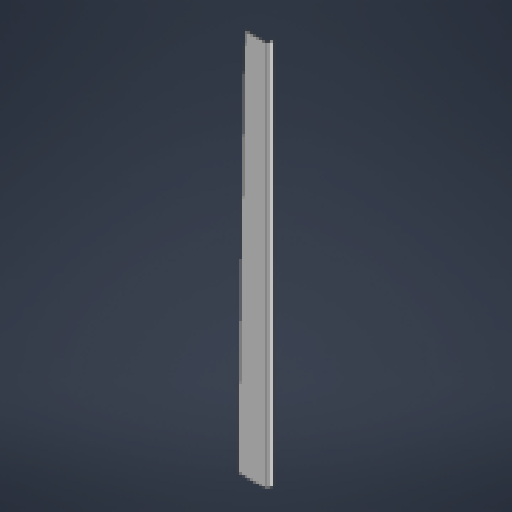
# Autodesk Inventor part: Part2_CPY_CPY
Saved by Autodesk Inventor 2026.2 (Build 302298000, 298)
## iProperties
Created: 2026-04-17
Part Number: Part2_CPY_CPY
Material: Generic
Document SubType Name: Sheet Metal
Designer: admin
Density: 1 g/cm^3
Sheet Metal Rule: Default
Appearance: Default
Author: admin
Autodesk Inventor part; units mm, degrees
ref_plane "YZ Plane" through (0, 0, 0) normal (1, 0, 0) x (0, 1, 0)
ref_plane "XZ Plane" through (0, 0, 0) normal (0, 1, 0) x (-1, 0, 0)
ref_plane "XY Plane" through (0, 0, 0) normal (0, 0, 1) x (1, 0, 0)
sketch "Sketch1" plane through (0, 0, 0) normal (0, 0, 1) x (1, 0, 0)
  line L0 (0, 0) -> (0, 1600)
  line L1 (0, 1600) -> (-106.3333, 1600)
  line L2 (-106.3333, 1600) -> (-134.2614, 0)
  line L3 (-134.2614, 0) -> (0, 0)
  line L4 (-107.206, 1550.0076) -> (-112.2052, 1550.0949)
  line L5 (-112.2052, 1550.0949) -> (-139.2622, 0)
  line L6 (-139.2622, 0) -> (-134.2614, 0)
  line L7 (-139.2622, 0) -> (-134.2614, 0) construction
  dimension "d0" = 1600
  dimension "d1" = 106.333
  dimension "d2" = 5
  dimension "d3" = 139.2622
  dimension "d4" = 0
  dimension "d6" = 50
  dimension "d17" = 89
  measures "d0" distance of L0.start L0.end
  measures "d2" distance of L4.start L4.end
  measures "d4" distance of L5.end L6.start
  measures "d6" distance from line of L1.end L4
  measures "d17" angle of L3 L2
extrude "Plate1" add sketch "Sketch1" along normal blind 3.048
sketch "Sketch2" plane through (-3.048, 0, 3.048) normal (1, 0, 0) x (0, 1, 0)
  line L0 (1600, 0) -> (0, 0)
  line L1 (0, 0) -> (0, -28)
  line L2 (0, -28) -> (1600, -28)
  line L3 (1600, -28) -> (1600, 0)
  constraints: 6 end point, 1 horizontal, 1 perpendicular, 1 vertical
edge flange "Flange1" height 28 angle 90 thickness 3.048 bend radius 3.048 thickness toward (1, 0, 0) relief straight relief width 3.048 relief depth 1.524 edges at (0, 800, 0) wall of the first edge with corners at (-3.048, 1600, 3.048) (-3.048, 0, 3.048) (-3.048, 0, -24.952) (-3.048, 1600, -24.952)
bend "Bend1"
corner "Corner1"
equation "\"d5\" = Thickness"
equation "\"d7\" = BendReliefWidth"
equation "\"d8\" = BendReliefDepth"
equation "\"d9\" = MinimumRemnant"
equation "\"d10\" = TransitionRadius"
equation "\"d13\" = BendRadius"
equation "\"d14\" = CornerReliefSize"
equation "\"d15\" = GapSize"
equation "\"d16\" = JacobiRadiusSize"
equation "\"BendRadius\" = Thickness"
equation "\"BendReliefWidth\" = Thickness"
equation "\"BendReliefDepth\" = 0.5 * Thickness"
equation "\"CornerReliefSize\" = 4 * Thickness"
equation "\"MinimumRemnant\" = 2 * Thickness"
equation "\"TransitionRadius\" = BendRadius"
equation "\"JacobiRadiusSize\" = BendRadius"
equation "\"GapSize\" = Thickness"
equation "\"Thickness\" = 3.048"
body "Solid1"
